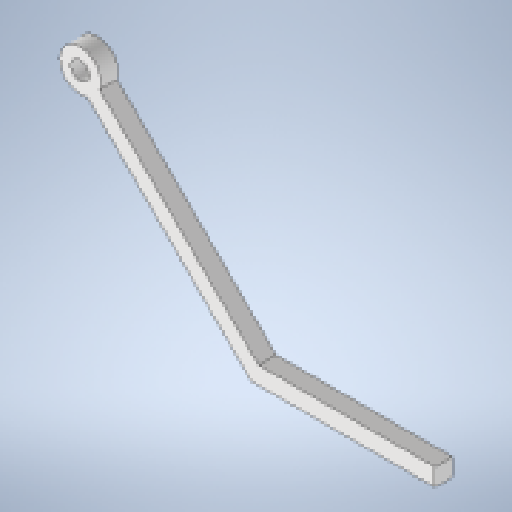
# Autodesk Inventor part: FrontLock
Saved by Autodesk Inventor 2025.1 (Build 291241000, 241)
## iProperties
Created: 2026-05-10
Part Number: FrontLock
Material: Generic
Document SubType Name: Modeling
Designer: User
Density: 1 g/cm^3
Appearance: Default
Author: User
Autodesk Inventor part; units mm, degrees
ref_plane "YZ Plane" through (0, 0, 0) normal (1, 0, 0) x (0, 1, 0)
ref_plane "XZ Plane" through (0, 0, 0) normal (0, 1, 0) x (-1, 0, 0)
ref_plane "XY Plane" through (0, 0, 0) normal (0, 0, 1) x (1, 0, 0)
sketch "Sketch1" plane through (0, 0, 0) normal (0, 0, 1) x (1, 0, 0)
  circle A0 centre (-6.4853, 1.4853) radius 1.5
  circle A1 centre (-6.4853, 1.4853) radius 1.6
  line L0 (4, 5) -> (-10, 5)
  line L1 (-10, 5) -> (-10, -7)
  line L2 (-3, 0) -> (-5, -2)
  circle A2 centre (-6.4853, 1.4853) radius 3.5147
  line L3 (54.1048, -60.4376) -> (54.1048, 0)
  line L4 (-6.4853, 1.4853) -> (54.1048, -59.1048)
  line L5 (-6.4853, 1.4853) -> (79.202, 1.4853) construction
  line L6 (-10, -7) -> (-5, -7)
  line L7 (-5, -2) -> (-3, 0)
  line L8 (-5, -2) -> (-3, 0)
  line L9 (-5, -7.5) -> (-10.5, -7.5)
  line L10 (-10.5, -7.5) -> (-10.5, 5.5)
  line L11 (-10.5, 5.5) -> (4, 5.5)
  line L12 (-2.6464, -0.3536) -> (-4.6464, -2.3536)
  circle A3 centre (-6.4853, 1.4853) radius 9.1072
  circle A4 centre (-6.4853, 1.4853) radius 9.8414
  line L13 (0.4736, -5.4736) -> (-0.587, -6.5343)
  line L14 (0.4736, -5.4736) -> (1.9736, -5.4736) construction
  line L15 (-0.587, -6.5343) -> (1.5343, -4.413)
  line L16 (23.8097, -28.8097) -> (24.8704, -27.7491)
  line L17 (1.5343, -4.413) -> (-0.587, -6.5343)
  line L18 (-0.587, -6.5343) -> (22.7491, -29.8704)
  line L19 (22.7491, -29.8704) -> (24.8704, -27.7491)
  line L20 (24.8704, -27.7491) -> (1.5343, -4.413)
  line L21 (-0.587, -6.5343) -> (1.5343, -4.413)
  line L22 (1.5343, -4.413) -> (-3.8267, 0.948)
  line L23 (-3.8267, 0.948) -> (-5.948, -1.1733)
  line L24 (-5.948, -1.1733) -> (-0.587, -6.5343)
  line L25 (22.7491, -29.8704) -> (54.1048, -29.8704)
  line L26 (54.1048, -29.8704) -> (54.1048, -26.8704)
  line L27 (54.1048, -26.8704) -> (22.7491, -26.8704)
  line L28 (22.7491, -26.8704) -> (22.7491, -29.8704)
  point P0 (0, 0)
  point P1 (-3.177, 0.2984)
  point P2 (-5.2984, -1.823)
  point P3 (23.9917, -26.8704)
extrude "Extrusion1" add sketch "Sketch1" along normal blind 3 contours A2 L22 L23 L24 | L22 L15 A4 | A4 L4 A3 L22 | A3 L4 A2 L22 | A4 L24 A3 L4 | L15 L20 L27 L28 L4 | L13 L24 A4 | L4 L28 L18 L13 | A2 L4 L23 L22 | L24 L23 L4 A2 | A2 L4 A3 L24 | L28 L27 L20 L16 L4 | L4 L19 L28 | L27 L3 L25 L4 L16 L20 | L4 L25 L19
sketch "Sketch2" plane through (0, 0, 0) normal (0, 0, -1) x (-1, 0, 0)
  line L0 (10, -7) -> (5, -7) projected
  line L1 (5.2984, -1.823) -> (-22.7491, -29.8704) projected
  arc A0 (5.2984, -1.823) -> (3.177, 0.2984) centre (6.4853, 1.4853) ccw projected
  line L2 (-23.9917, -26.8704) -> (3.177, 0.2984) projected
  line L3 (-54.1048, -26.8704) -> (-23.9917, -26.8704) projected
  line L4 (-54.1048, -29.8704) -> (-54.1048, -26.8704) projected
  line L5 (-22.7491, -29.8704) -> (-54.1048, -29.8704) projected
  circle A1 centre (6.4853, 1.4853) radius 1.6 projected
  circle A2 centre (6.4853, 1.4853) radius 9.1844
  circle A3 centre (6.4853, 1.4853) radius 9.6844
  point P0 (0, 0)
  point P1 (-1.3406, -4.2193)
  point P2 (0.7807, -6.3406)
  dimension "d11" = 0.5
  constraints: 1 centre point, 1 coincident, 3 other
extrude "Extrusion2" cut sketch "Sketch2" against normal blind 0.2 contours L1 A2 L2 A0 | L1 A3 L2 A2 picked at (2.707, -2.0563) picked at (-0.8925, -4.2416)
sketch "Sketch3" plane through (0, 0, 0) normal (0, 0, -1) x (-1, 0, 0)
  arc A0 (-1.3406, -4.2193) -> (0.7807, -6.3406) centre (6.4853, 1.4853) ccw projected
  line L0 (-23.9917, -26.8704) -> (-1.3406, -4.2193) projected
  line L1 (-54.1048, -26.8704) -> (-23.9917, -26.8704) projected
  line L2 (-54.1048, -29.8704) -> (-54.1048, -26.8704) projected
  line L3 (-22.7491, -29.8704) -> (-54.1048, -29.8704) projected
  line L4 (0.7807, -6.3406) -> (-22.7491, -29.8704) projected
  point P0 (0, 0)
ref_plane "Work Plane1" through (-10, -7, -78.1802) normal (0, 0, -1) x (0, 1, 0)
extrude "Extrusion3" add sketch "Sketch3" along normal up to surface (78.1802 mm away)
sketch "Sketch4" plane through (54.1048, -29.8704, -78.1802) normal (0, 0, -1) x (-1, 0, 0)
  line L0 (30.113, 3) -> (52.7641, 25.6511) projected
  line L1 (0, 3) -> (30.113, 3) projected
  line L2 (0, 0) -> (0, 3) projected
  line L3 (31.3557, 0) -> (0, 0) projected
  line L4 (54.8854, 23.5298) -> (31.3557, 0) projected
  arc A0 (52.7641, 25.6511) -> (54.8854, 23.5298) centre (60.59, 31.3557) ccw projected
  point P0 (54.1048, 29.8704)
extrude "Extrusion4" add sketch "Sketch4" along normal blind 0.2
sketch "Sketch6" plane through (54.1048, -29.8704, -78.3802) normal (0, 0, -1) x (-1, 0, 0)
  line L0 (59.4031, 28.0474) -> (31.3557, 0) projected
  line L1 (31.3557, 0) -> (0, 0) projected
  line L2 (0, 0) -> (0, 3) projected
  line L3 (0, 3) -> (30.113, 3) projected
  line L4 (30.113, 3) -> (57.2818, 30.1688) projected
  arc A0 (59.4031, 28.0474) -> (57.2818, 30.1688) centre (60.59, 31.3557) ccw projected
  circle A1 centre (60.59, 31.3557) radius 1.6 projected
  point P0 (54.1048, 29.8704)
extrude "Extrusion5" add sketch "Sketch6" along normal blind 2.8
sketch "Sketch7" plane through (22.7491, -29.8704, 3) normal (0, -1, 0) x (1, 0, 0)
  line L0 (9.1991, -15.9198) -> (19.1991, -25.9198) projected
  line L1 (-21.5775, 14.8568) -> (9.1991, -15.9198) projected
  line L2 (19.1991, -57.9373) -> (9.1991, -67.9373) projected
  line L3 (-21.5775, -98.7139) -> (9.1991, -67.9373) projected
  line L4 (0, -84.1802) -> (-28.0474, -84.1802) projected
  line L5 (31.3557, -84.1802) -> (0, -84.1802) projected
  line L6 (31.3557, -84.1802) -> (31.3557, 0) projected
  line L7 (0, 0) -> (31.3557, 0) projected
  line L8 (-28.0474, 0) -> (0, 0) projected
  line L9 (19.1991, -25.9198) -> (29.7682, -36.4889) projected
  line L10 (19.1991, -57.9373) -> (29.7439, -47.3925) projected
  line L11 (19.1991, -25.9198) -> (19.1991, -57.9373)
  line L12 (19.1991, -25.9198) -> (51.2166, -25.9198) construction
  line L13 (29.7682, -36.4889) -> (29.7439, -47.3925)
  line L14 (29.7439, -47.3925) -> (8.744, -47.3457)
  line L15 (8.744, -47.3457) -> (8.7683, -36.4421)
  line L16 (8.7683, -36.4421) -> (29.7682, -36.4889)
  line L17 (-22.9917, 13.4426) -> (7.7849, -17.334)
  line L18 (7.7849, -17.334) -> (17.7849, -27.334)
  line L19 (17.7849, -27.334) -> (28.354, -37.9031)
  line L20 (-22.9917, -97.2997) -> (7.7849, -66.5231)
  line L21 (7.7849, -66.5231) -> (17.7849, -56.5231)
  line L22 (17.7849, -56.5231) -> (28.3297, -45.9783)
  point P0 (-22.7491, -3)
  point P1 (-9.5491, 0)
  point P2 (19.1991, -28.7482)
  point P3 (19.1991, -36.4653)
  point P4 (19.1991, -47.369)
  point P5 (19.1991, -55.1089)
  point P6 (-9.8723, -84.1802)
  dimension "d20" = 90
  dimension "d21" = 21
  dimension "d22" = 2
  dimension "d23" = 2
  constraints: 24 end point, 2 parallel, 2 perpendicular, 1 horizontal, 1 point on line, 4 other
  measures "d20" angle of L11 L12
  measures "d21" distance of L10.end L14.end
  measures "d22" distance between parallel lines of L1 L17
  measures "d23" distance between parallel lines of L3 L20
extrude "Extrusion6" cut sketch "Sketch7" against normal blind 21
chamfer "Chamfer1" distance 2 angle 45 2 edges at (41.9482, -28.3704, -33.4653) (41.9482, -28.3704, -44.369)
fillet "Fillet1" radius 2 12 edges at (31.5174, -28.3704, -33.4421) (39.9482, -28.3704, -33.4609) (41.9482, -28.3704, -31.4653) (31.493, -28.3704, -44.3457) (39.9482, -28.3704, -44.3645) (41.9482, -28.3704, -46.369) (41.9482, -28.3704, -52.1089) (41.9482, -28.3704, -25.7482) (13.2, -18.2, 3) (12.8768, -17.8768, -81.1802) (22.7491, -29.8704, -38.9285) (23.9917, -26.8704, -38.9285)
sketch "Sketch8" plane through (0, 0, 3) normal (0, 0, 1) x (1, 0, 0)
  arc A0 (-3.177, 0.2984) -> (-5.2984, -1.823) centre (-6.4853, 1.4853) ccw projected
  line L0 (-5.2984, -1.823) -> (12.3716, -19.4929) projected
  arc A1 (-0.7807, -6.3406) -> (1.3406, -4.2193) centre (-6.4853, 1.4853) ccw projected
  line L1 (3.6787, -13.6493) -> (-13.0339, 3.0633)
  line L2 (-0.7807, -6.3406) -> (-2.2053, -7.7653)
  line L3 (-0.7807, -6.3406) -> (1.234, -6.3406) construction
  line L4 (-0.7807, -6.3406) -> (-5.2984, -1.823) projected
  line L5 (-0.7807, -6.3406) -> (-2.2053, -7.7653)
  line L6 (-2.2053, -7.7653) -> (-0.7805, -9.1901)
  line L7 (-0.7805, -9.1901) -> (0.6441, -7.7655)
  line L8 (0.6441, -7.7655) -> (-0.7807, -6.3406)
  point P0 (0, 0)
  dimension "d30" = 135
  dimension "d31" = 2.015
  constraints: 14 end point, 3 parallel, 1 equal length, 1 horizontal, 1 perpendicular, 1 point on line, 1 tangent
  measures "d30" angle of L2 L3
  measures "d31" distance of L6.end L2.end
extrude "Extrusion7" add sketch "Sketch8" against normal up to surface (84.1802 mm away) contours L2 L0 L7 L1
sketch "Sketch9" plane through (0, 0, 3) normal (0, 0, 1) x (1, 0, 0)
  line L0 (-5.2984, -1.823) -> (-0.7807, -6.3406) projected
  line L1 (-0.7807, -6.3406) -> (-2.2053, -7.7653) projected
  arc A0 (-3.177, 0.2984) -> (-5.2984, -1.823) centre (-6.4853, 1.4853) ccw projected
  line L2 (-2.2053, -7.7653) -> (-8.9706, -1)
  point P0 (0, 0)
  constraints: 2 end point, 1 point on circle, 1 tangent
extrude "Extrusion8" add sketch "Sketch9" against normal up to surface (2.8 mm away)
sketch "Sketch10" plane through (54.1048, -29.8704, -81.1802) normal (0, 0, -1) x (-1, 0, 0)
  line L0 (54.8854, 23.5298) -> (56.3101, 22.1051) projected
  line L1 (54.8854, 23.5298) -> (59.4031, 28.0474) projected
  arc A0 (59.4031, 28.0474) -> (57.2818, 30.1688) centre (60.59, 31.3557) ccw projected
  line L2 (63.0753, 28.8704) -> (56.3101, 22.1051) projected
  point P0 (54.1048, 29.8704)
extrude "Extrusion9" add sketch "Sketch10" against normal up to surface (2.8 mm away)
sketch "Sketch11" plane through (22.1633, -29.2846, -5.9633) normal (-0.7071068, -0.7071068, 0) x (-0.7071068, 0.7071068, 0)
  line L0 (30.4327, -8.9633) -> (30.4327, 75.2169) projected
  line L1 (32.4477, -6.1633) -> (32.4477, 72.4169) projected
  line L2 (32.4477, 72.4169) -> (32.4477, -6.1633) projected
  line L3 (30.4327, 49.5073) -> (32.4477, 49.5073)
  line L4 (32.4477, 49.5073) -> (32.4477, 58.5073)
  line L5 (32.4477, 58.5073) -> (30.4327, 58.5073)
  line L6 (30.4327, 58.5073) -> (30.4327, 49.5073)
  point P0 (36.3792, -5.9633)
  point P1 (30.4327, 58.5073)
  dimension "d38" = 9
  constraints: 8 end point, 2 parallel, 2 point on line, 1 horizontal, 1 perpendicular
  measures "d38" distance of L4.end L3.end
extrude "Extrusion10" cut sketch "Sketch11" along normal blind 10
sketch "Sketch13" plane through (22.1633, -29.2846, -5.9633) normal (-0.7071068, -0.7071068, 0) x (-0.7071068, 0.7071068, 0)
  line L0 (25.7327, 40.7255) -> (25.7327, 49.2073)
  line L1 (26.2327, 49.7073) -> (25.7327, 49.2073)
  line L2 (26.2327, 49.7073) -> (35.6319, 49.7073)
  line L3 (29.7327, 40.2255) -> (26.2327, 40.2255)
  line L4 (25.7327, 40.7255) -> (26.2327, 40.2255)
  line L5 (30.4327, -8.9633) -> (30.4327, 49.5073)
  line L6 (30.2327, 20.272) -> (30.2327, 39.7255)
  line L7 (30.2327, 39.7255) -> (29.7327, 40.2255)
  line L8 (35.6319, 49.2073) -> (26.4398, 49.2073)
  line L9 (26.4398, 49.2073) -> (26.2327, 49.0002)
  line L10 (26.2327, 49.0002) -> (26.2327, 40.9326)
  line L11 (26.2327, 40.9326) -> (26.4398, 40.7255)
  line L12 (26.4398, 40.7255) -> (29.9398, 40.7255)
  line L13 (29.9398, 40.7255) -> (30.7327, 39.9326)
  line L14 (30.7327, 39.9326) -> (30.7327, 20.272)
  line L15 (26.4398, 40.7255) -> (30.4327, 40.7255)
  point P0 (36.3792, -5.9633)
  point P1 (30.4327, 49.2073)
extrude "Extrusion11" add sketch "Sketch13" along normal up to surface (2.0147 mm away) contours L15 L12 L11 L10 L9 L8 L5
sketch "Sketch14" plane through (-8.9706, -1, 3) normal (-0.7071068, -0.7071068, 0) x (-0.7071068, 0.7071068, 0)
  line L0 (-15.7825, 49.8959) -> (-15.7825, 57.9635) projected
  line L1 (-9.5675, 2.8) -> (-9.5675, 58.4706) projected
  line L2 (-15.7825, 53.9297) -> (-9.5675, 53.9297)
  circle A0 centre (-12.675, 53.9297) radius 1.5
  point P0 (-5.636, 3)
  dimension "d44" = 3
  constraints: 2 end point, 2 midpoint, 1 centre point, 1 perpendicular, 1 point on line
  measures "d44" diameter of A0
extrude "Extrusion12" cut sketch "Sketch14" against normal blind 10
sketch "Sketch15" plane through (22.1633, -29.2846, -5.9633) normal (-0.7071068, -0.7071068, 0) x (-0.7071068, 0.7071068, 0)
  circle A0 centre (25.2327, 20.272) radius 1.6 projected
  circle A1 centre (25.2327, 20.272) radius 1.5
  point P0 (36.3792, -5.9633)
  dimension "d47" = 3
  constraints: 1 centre point, 1 coincident
  measures "d47" diameter of A1
extrude "Extrusion13" cut sketch "Sketch15" against normal blind 10 contours A1
sketch "Sketch16" plane through (0.6441, -7.7655, -55.4706) normal (0, 0, -1) x (-0.7071068, -0.7071068, 0)
  line L0 (0, -4.2) -> (2.5, -4.2) projected
  line L1 (0, 7.215) -> (0, -4.2) projected
  line L2 (0, 7.215) -> (0.4842, 7.215) projected
  line L3 (0.4842, 7.215) -> (2.5, 5.1992) projected
  line L4 (2.5, -4.2) -> (2.5, 5.1992) projected
  line L5 (0, 2.015) -> (2.0147, 2.015) projected
  line L6 (2.5, -4.2) -> (2.5, 5.1992) projected
  line L7 (2.0147, 0) -> (0, 0) projected
  line L8 (2.0147, 2.015) -> (2.0147, 0) projected
  point P0 (-5.0355, 5.9465)
extrude "Extrusion14" cut sketch "Sketch16" against normal up to surface (0.3 mm away) contours L1 L5 L8 L7
chamfer "Chamfer2" distance 1 angle 45 1 edges at (-0.0682, -8.4778, -64.4706)
sketch "Sketch17" plane through (0, 0, 3) normal (0, 0, 1) x (1, 0, 0)
  arc A0 (-3.177, 0.2984) -> (-8.9706, -1) centre (-6.4853, 1.4853) ccw projected
  line L0 (12.3716, -15.2502) -> (-3.177, 0.2984) projected
  line L1 (12.3716, -15.2502) -> (12.3716, -19.4929) projected
  line L2 (12.3716, -19.4929) -> (12.3716, -1.59)
  line L3 (16.6607, -16.6901) -> (-8.9996, 8.9701)
  point P0 (0, 0)
  point P1 (12.3716, -12.401)
  point P2 (-4, 3.9706)
  constraints: 4 end point, 1 parallel, 1 point on line, 1 tangent
extrude "Extrusion15" add sketch "Sketch17" against normal up to surface (2.8 mm away)
sketch "Sketch18" plane through (54.1048, -29.8704, -81.1802) normal (0, 0, -1) x (-1, 0, 0)
  line L0 (57.2818, 30.1688) -> (42.0564, 14.9433) projected
  line L1 (41.7332, 17.4694) -> (58.1048, 33.841) projected
  line L2 (40.6422, 13.5291) -> (42.0564, 14.9433) projected
  line L3 (41.7332, 14.6202) -> (41.7332, 17.4694) projected
  arc A0 (63.0753, 28.8704) -> (57.2818, 30.1688) centre (60.59, 31.3557) ccw projected
  point P0 (54.1048, 29.8704)
extrude "Extrusion16" add sketch "Sketch18" against normal up to surface (2.8 mm away)
sketch "Sketch19" plane through (0, 0, 3) normal (0, 0, 1) x (1, 0, 0)
  line L0 (-0.7805, -9.1901) -> (0.6441, -7.7655) projected
  line L1 (0.6441, -7.7655) -> (12.3716, -19.4929) projected
  line L2 (0.6441, -7.7655) -> (2.069, -9.1903)
  line L3 (0.6441, -7.7655) -> (2.6591, -7.7655) construction
  line L4 (2.069, -9.1903) -> (-0.7805, -9.1901)
  point P0 (0, 0)
  dimension "d59" = 2.015
  dimension "d60" = 45
  constraints: 6 end point, 1 equal length, 1 horizontal, 1 point on line
  measures "d59" distance of L0.end L2.end
  measures "d60" angle of L2 L3
ref_plane "Work Plane2" through (-5.3769, -31.2414, -20.7353) normal (0, 0, 1) x (0.7071068, 0.7071068, 0)
extrude "Extrusion17" add sketch "Sketch19" against normal up to surface (23.7353 mm away)
equation "\"d24\" = d21"
equation "\"d32\" = d21"
body "Solid1"
